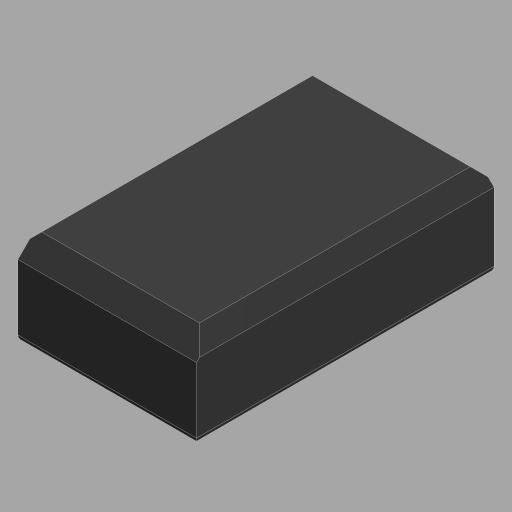
# Autodesk Inventor part: stone
Saved by Autodesk Inventor 2023 (Build 270158000, 158)
## iProperties
Created: 2023-08-01
Part Number: stone
Material: Rubber, Silicone
Document SubType Name: Modeling
Designer: Callan Littlejohn
Density: 1.25 g/cm^3
Appearance: Rubber - Black
Author: Callan Littlejohn
Autodesk Inventor part; units mm, degrees
ref_plane "YZ Plane" through (0, 0, 0) normal (1, 0, 0) x (0, 1, 0)
ref_plane "XZ Plane" through (0, 0, 0) normal (0, 1, 0) x (-1, 0, 0)
ref_plane "XY Plane" through (0, 0, 0) normal (0, 0, 1) x (1, 0, 0)
sketch "Sketch1" plane through (0, 0, 0) normal (0, 1, 0) x (-1, 0, 0)
  line L0 (20.6226, 45.3307) -> (-39.3774, 45.3307)
  line L1 (-39.3774, 45.3307) -> (-39.3774, -54.6693)
  line L2 (-39.3774, -54.6693) -> (20.6226, -54.6693)
  line L3 (20.6226, -54.6693) -> (20.6226, 45.3307)
  point P0 (0, 0)
  dimension "d0" = 100
  dimension "d1" = 60
  constraints: 8 end point, 2 parallel, 1 horizontal, 1 perpendicular
  measures "d0" distance of L2.end L0.start
  measures "d1" distance of L1.end L2.end
extrude "Extrusion1" add sketch "Sketch1" along normal blind 30
chamfer "Chamfer1" distance 5 angle 45 1 edges at (39.3774, 30, -4.6693)
chamfer "Chamfer2" distance 6 angle 45 1 edges at (6.8774, 30, 45.3307)
chamfer "Chamfer3" distance 3 angle 45 1 edges at (6.8774, 30, -54.6693)
chamfer "Chamfer4" distance 2 angle 45 1 edges at (-20.6226, 30, -6.1693)
fillet "Fillet1" radius 2 2 edges at (39.3774, 0, -4.6693) (9.3774, 0, 45.3307)
body "Solid1"
